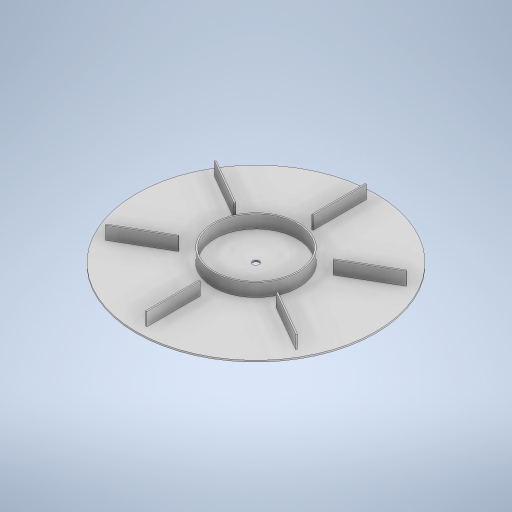
# Autodesk Inventor part: Plate
Saved by Autodesk Inventor 2024 (Build 280153000, 153)
## iProperties
Created: 2023-12-05
Part Number: Plate
Material: Generic
Document SubType Name: Modeling
Designer: 96279
Density: 1 g/cm^3
Appearance: Default
Author: 96279
Autodesk Inventor part; units mm, degrees
ref_plane "YZ Plane" through (0, 0, 0) normal (1, 0, 0) x (0, 1, 0)
ref_plane "XZ Plane" through (0, 0, 0) normal (0, 1, 0) x (-1, 0, 0)
ref_plane "XY Plane" through (0, 0, 0) normal (0, 0, 1) x (1, 0, 0)
sketch "Sketch4" plane through (0, 0, 0) normal (0, 1, 0) x (-1, 0, 0)
  circle A0 centre (0, 0) radius 32.5
  line L0 (85.3525, 23.3053) -> (40.3525, 23.3053)
  line L1 (40.3525, 23.3053) -> (40.3525, -21.6947)
  line L2 (40.3525, -21.6947) -> (85.3525, -21.6947)
  line L3 (85.3525, -21.6947) -> (85.3525, 23.3053)
  line L4 (22.4932, 85.5701) -> (-0.0068, 46.5989)
  line L5 (-0.0068, 46.5989) -> (38.9644, 24.0989)
  line L6 (38.9644, 24.0989) -> (61.4644, 63.0701)
  line L7 (61.4644, 63.0701) -> (22.4932, 85.5701)
  line L8 (-62.8593, 62.2648) -> (-40.3593, 23.2936)
  line L9 (-40.3593, 23.2936) -> (-1.3881, 45.7936)
  line L10 (-1.3881, 45.7936) -> (-23.8881, 84.7648)
  line L11 (-23.8881, 84.7648) -> (-62.8593, 62.2648)
  line L12 (-85.3525, -23.3053) -> (-40.3525, -23.3053)
  line L13 (-40.3525, -23.3053) -> (-40.3525, 21.6947)
  line L14 (-40.3525, 21.6947) -> (-85.3525, 21.6947)
  line L15 (-85.3525, 21.6947) -> (-85.3525, -23.3053)
  line L16 (-22.4932, -85.5701) -> (0.0068, -46.5989)
  line L17 (0.0068, -46.5989) -> (-38.9644, -24.0989)
  line L18 (-38.9644, -24.0989) -> (-61.4644, -63.0701)
  line L19 (-61.4644, -63.0701) -> (-22.4932, -85.5701)
  line L20 (62.8593, -62.2648) -> (40.3593, -23.2936)
  line L21 (40.3593, -23.2936) -> (1.3881, -45.7936)
  line L22 (1.3881, -45.7936) -> (23.8881, -84.7648)
  line L23 (23.8881, -84.7648) -> (62.8593, -62.2648)
  circle A1 centre (0, 0) radius 91
  line L24 (0, -32.5) -> (0, -91)
  dimension "d5" = 65
  dimension "d12" = 182
  dimension "d6" = 45
  dimension "d7" = 45
  dimension "d10" = 360
  constraints: 50 end point, 2 coincident, 2 parallel, 2 vertical alignment, 1 horizontal, 1 perpendicular, 1 vertical, 53 other
  measures "d6" distance of L2.end L0.start
  measures "d7" distance of L0.start L0.end
extrude "Extrusion2" add sketch "Sketch4" against normal blind 1.2 contours A0 | A1 | L17 L16 L24 | L24 L16 L19 L18 L17 | L3 L2 L1 L0 | L7 L6 L5 L4 | L11 L10 L9 L8 | L15 L14 L13 L12 | L23 L22 L21 L20
sketch "Sketch6" plane through (0, 0, 0) normal (0, 1, 0) x (1, 0, 0)
  circle A0 centre (0, 0) radius 42.5
  circle A1 centre (0, 0) radius 91 projected
  line L0 (-0.7102, 83.7173) -> (0.2898, 83.7173)
  line L1 (0.2898, 83.7173) -> (0.2898, 43.1226)
  line L2 (0.2898, 43.1226) -> (-0.7102, 43.1226)
  line L3 (-0.7102, 43.1226) -> (-0.7102, 83.7173)
  dimension "d15" = 85
  dimension "d16" = 1
  constraints: 8 end point, 2 parallel, 1 centre point, 1 coincident, 1 horizontal, 1 perpendicular
  measures "d15" diameter of A0
  measures "d16" distance of L1.end L2.end
extrude "Extrusion3" add sketch "Sketch6" along normal blind 10 contours L0 L1 L2 L3
pattern_circular "Circular Pattern1" count 6 over 360 about axis through (0, -10, 0) along (0, 1, 0) of "Extrusion3"
sketch "Sketch7" plane through (0, 0, 0) normal (0, 1, 0) x (1, 0, 0)
  circle A0 centre (0, 0) radius 32.5
  dimension "d24" = 65
  constraints: 1 centre point, 1 coincident
  measures "d24" diameter of A0
extrude "Extrusion4" add sketch "Sketch7" along normal blind 10
sketch "Sketch12" plane through (0, 10, 0) normal (0, 1, 0) x (1, 0, 0)
  point P0 (0, 0)
  point P1 (0, 0)
  constraints: 1 coincident
hole "Hole3" at (0, 10, 0) direction (0, -1, 0) diameter 63 depth 10
sketch "Sketch13" plane through (0, 0, 0) normal (0, 1, 0) x (1, 0, 0)
  point P0 (0, 0)
  point P1 (0, 0)
  constraints: 1 coincident
hole "Hole4" at (0, 0, 0) direction (0, -1, 0) diameter 5 depth 2
body "Solid2"
